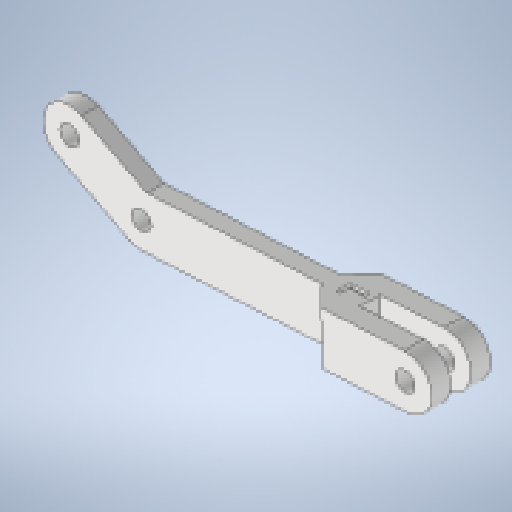
# Autodesk Inventor part: GripperShaftLeft
Saved by Autodesk Inventor 2025.1 (Build 291241000, 241)
## iProperties
Created: 2026-05-06
Part Number: GripperShaftLeft
Material: Generic
Document SubType Name: Modeling
Designer: User
Density: 1 g/cm^3
Appearance: Default
Author: User
## iProperties of the stored document GripperShaftLeft_3DPrint.ipt
Created: 2026-05-06
Part Number: GripperShaftLeft_3DPrint
Material: Generic
Document SubType Name: Modeling
Designer: User
Density: 1 g/cm^3
Appearance: Default
Author: User
Autodesk Inventor part; units mm, degrees
ref_plane "YZ Plane" through (0, 0, 0) normal (1, 0, 0) x (0, 1, 0)
ref_plane "XZ Plane" through (0, 0, 0) normal (0, 1, 0) x (-1, 0, 0)
sketch "Sketch1" plane through (0, 0, 0) normal (0, 0, 1) x (1, 0, 0)
  line L0 (-26.293304, 15.205533) -> (-26.696935, 23.195344)
  line L1 (-26.696935, 23.195344) -> (-13.921595, 23.840732)
  arc A0 (-13.517964, 15.85092) -> (-13.921595, 23.840732) centre (-13.719779, 19.845826) ccw
  line L2 (-13.517964, 15.85092) -> (-26.293304, 15.205533)
  circle A1 centre (-13.719779, 19.845826) radius 1.5
  point P0 (0, 0)
sketch "Sketch1 outline for Extrusion1" plane through (0, 0, 0) normal (0, 0, 1) x (1, 0, 0)
  arc A0 (-13.517964, 15.85092) -> (-13.921595, 23.840732) centre (-13.719779, 19.845826) ccw
  line L0 (-26.293304, 15.205533) -> (-13.517964, 15.85092)
  line L1 (-13.921595, 23.840732) -> (-26.696935, 23.195344)
  line L2 (-26.696935, 23.195344) -> (-26.293304, 15.205533)
  circle A1 centre (-13.719779, 19.845826) radius 1.5
extrude "Extrusion1" add sketch "Sketch1 outline for Extrusion1" along normal blind 3
sketch "Sketch2" plane through (0, 0, 0) normal (0, 0, -1) x (-1, 0, 0)
  line L0 (23.700756, 23.346705) -> (23.297124, 15.356894)
  line L1 (26.696935, 23.195344) -> (26.293304, 15.205533)
  line L2 (13.921595, 23.840732) -> (26.696935, 23.195344)
  arc A0 (13.921595, 23.840732) -> (13.517964, 15.85092) centre (13.719779, 19.845826) ccw
  line L3 (26.293304, 15.205533) -> (13.517964, 15.85092)
  line L4 (26.696935, 23.195344) -> (26.293304, 15.205533)
  circle A1 centre (13.719779, 19.845826) radius 1.5
  point P0 (0, 0)
sketch "Sketch2 outline for Extrusion2" plane through (0, 0, 0) normal (0, 0, -1) x (-1, 0, 0)
  line L0 (23.297124, 15.356894) -> (26.293304, 15.205533)
  line L1 (23.700756, 23.346705) -> (23.297124, 15.356894)
  line L2 (26.696935, 23.195344) -> (23.700756, 23.346705)
  line L3 (26.293304, 15.205533) -> (26.696935, 23.195344)
extrude "Extrusion2" add sketch "Sketch2 outline for Extrusion2" along normal blind 3.1
sketch "Sketch3" plane through (0, 0, -3.1) normal (0, 0, -1) x (-1, 0, 0)
  line L0 (13.921595, 23.840732) -> (26.696935, 23.195344)
  line L1 (26.696935, 23.195344) -> (26.293304, 15.205533)
  line L2 (26.293304, 15.205533) -> (13.517964, 15.85092)
  arc A0 (13.921595, 23.840732) -> (13.517964, 15.85092) centre (13.719779, 19.845826) ccw
  circle A1 centre (13.719779, 19.845826) radius 1.5
  point P0 (0, 0)
sketch "Sketch3 outline for Extrusion3" plane through (0, 0, -3.1) normal (0, 0, -1) x (-1, 0, 0)
  arc A0 (13.921595, 23.840732) -> (13.517964, 15.85092) centre (13.719779, 19.845826) ccw
  line L0 (26.696935, 23.195344) -> (13.921595, 23.840732)
  line L1 (13.517964, 15.85092) -> (26.293304, 15.205533)
  line L2 (26.293304, 15.205533) -> (26.696935, 23.195344)
  circle A1 centre (13.719779, 19.845826) radius 1.5
extrude "Extrusion3" add sketch "Sketch3 outline for Extrusion3" along normal blind 3
sketch "Sketch4" plane through (0, 0, 0) normal (0, 0, -1) x (-1, 0, 0)
  arc A0 (57.453567, 13.631371) -> (57.857198, 21.621182) centre (57.655383, 17.626276) ccw
  line L0 (57.453567, 13.631371) -> (29.389355, 15.049125)
  line L1 (29.792987, 23.038937) -> (29.389355, 15.049125)
  line L2 (29.792987, 23.038937) -> (57.857198, 21.621182)
  circle A1 centre (57.655383, 17.626276) radius 1.5
  line L3 (29.389355, 15.049125) -> (26.293304, 15.205533)
  line L4 (26.696935, 23.195344) -> (26.293304, 15.205533)
  line L5 (26.696935, 23.195344) -> (29.792987, 23.038937)
  line L6 (29.792987, 23.038937) -> (29.389355, 15.049125)
  circle A2 centre (68.688702, 23.388615) radius 1.5
  arc A3 (70.540437, 19.843043) -> (66.836967, 26.934186) centre (68.688702, 23.388615) ccw
  line L7 (59.507118, 14.080705) -> (70.540437, 19.843043)
  arc A4 (57.453567, 13.631371) -> (57.857198, 21.621182) centre (57.655383, 17.626276) ccw
  line L8 (56.769238, 21.676144) -> (66.836967, 26.934186)
  point P0 (0, 0)
  dimension "d18" = 8
  constraints: 6 end point, 5 point on circle, 4 tangent, 2 centre point, 2 coincident, 1 concentric, 1 point on line
  measures "d18" diameter of A3
sketch "Sketch4 outline for Extrusion4" plane through (0, 0, 0) normal (0, 0, -1) x (-1, 0, 0)
  line L0 (26.696935, 23.195344) -> (26.293304, 15.205533)
  line L1 (26.293304, 15.205533) -> (57.453567, 13.631371)
  arc A0 (57.453567, 13.631371) -> (59.507118, 14.080705) centre (57.655383, 17.626276) ccw
  line L2 (59.507118, 14.080705) -> (70.540437, 19.843043)
  arc A1 (70.540437, 19.843043) -> (66.836967, 26.934186) centre (68.688702, 23.388615) ccw
  line L3 (66.836967, 26.934186) -> (56.769238, 21.676144)
  line L4 (56.769238, 21.676144) -> (26.696935, 23.195344)
  circle A2 centre (57.655383, 17.626276) radius 1.5
  circle A3 centre (68.688702, 23.388615) radius 1.5
extrude "Extrusion4" add sketch "Sketch4 outline for Extrusion4" along normal blind 3
chamfer "Chamfer1" distance 3 angle 45 1 edges at (-26.4951, 19.2004, 0)
chamfer "Chamfer2" distance 3.1 angle 45 1 edges at (-26.4951, 19.2004, -3)
ref_plane "Work Plane1" through (-62.942605, 1.312432, -0.38873) normal (0, 0, -1) x (-0.0504539, 0.9987264, 0)
sketch "Sketch6" plane through (0, 0, 0) normal (0, 0, 1) x (1, 0, 0)
  line L0 (-57.453567, 13.631371) -> (-48.265284, 14.095547)
  arc A0 (-57.857198, 21.621182) -> (-57.453567, 13.631371) centre (-57.655383, 17.626276) ccw
  line L1 (-29.693114, 23.043982) -> (-57.857198, 21.621182)
  line L2 (-29.693114, 23.043982) -> (-48.265284, 14.095547)
  circle A1 centre (-57.655383, 17.626276) radius 1.5
  point P0 (0, 0)
sketch "Sketch6 outline for Extrusion5" plane through (0, 0, 0) normal (0, 0, 1) x (1, 0, 0)
  line L0 (-29.693114, 23.043982) -> (-57.857198, 21.621182)
  line L1 (-48.265284, 14.095547) -> (-29.693114, 23.043982)
  arc A0 (-57.857198, 21.621182) -> (-57.453567, 13.631371) centre (-57.655383, 17.626276) ccw
  line L2 (-57.453567, 13.631371) -> (-48.265284, 14.095547)
  circle A1 centre (-57.655383, 17.626276) radius 1.5
extrude "Extrusion5" cut sketch "Sketch6 outline for Extrusion5" against normal up to surface (0.38873 mm away)
sketch "Sketch7" plane through (-13.921595, 23.840732, 3) normal (-0.0504539, 0.9987264, 0) x (0.9987264, 0.0504539, 0)
  line L0 (-10.748057, 5.806776) -> (-10.748057, 3.406816) construction
  line L1 (-10.748057, 3.406816) -> (-13.798057, 3.406816) construction
  line L2 (-13.798057, 3.406816) -> (-13.798057, 5.806776) construction
  line L3 (-13.798057, 5.806776) -> (-10.748057, 5.806776) construction
  line L4 (-13.798057, 3.456249) -> (-13.798057, 5.490406)
  line L5 (-13.798057, 5.490406) -> (-10.748057, 5.490406)
  line L6 (-10.748057, 5.490406) -> (-10.748057, 4.724199)
  line L7 (-10.748057, 4.724199) -> (-13.217222, 4.724199)
  line L8 (-13.217222, 4.724199) -> (-13.217222, 3.456249)
  line L9 (-13.217222, 3.456249) -> (-13.798057, 3.456249)
  point P0 (12.701006, 3)
  constraints: 2 other
sketch "Sketch7 outline for Emboss1" plane through (-13.921595, 23.840732, 3) normal (-0.0504539, 0.9987264, 0) x (0.9987264, 0.0504539, 0)
  line L0 (-13.798057, 3.456249) -> (-13.798057, 5.490406)
  line L1 (-13.798057, 5.490406) -> (-10.748057, 5.490406)
  line L2 (-10.748057, 5.490406) -> (-10.748057, 4.724199)
  line L3 (-10.748057, 4.724199) -> (-13.217222, 4.724199)
  line L4 (-13.217222, 4.724199) -> (-13.217222, 3.456249)
  line L5 (-13.217222, 3.456249) -> (-13.798057, 3.456249)
emboss "Emboss1" sketch "Sketch7 outline for Emboss1" operation cut depth 0.5 direction (0.0504539, -0.9987264, 0)
sketch "Sketch8" plane through (0, 0, 0) normal (0, 0, 1) x (1, 0, 0)
  line L0 (-57.857198, 21.621182) -> (-56.769238, 21.676144)
  line L1 (-66.836967, 26.934186) -> (-56.769238, 21.676144)
  arc A0 (-66.836967, 26.934186) -> (-70.540437, 19.843043) centre (-68.688702, 23.388615) ccw
  line L2 (-59.507118, 14.080705) -> (-70.540437, 19.843043)
  arc A1 (-57.857198, 21.621182) -> (-59.507118, 14.080705) centre (-57.655383, 17.626276) ccw
  circle A2 centre (-68.688702, 23.388615) radius 1.5
  point P0 (0, 0)
sketch "Sketch8 outline for Extrusion6" plane through (0, 0, 0) normal (0, 0, 1) x (1, 0, 0)
  arc A0 (-59.507118, 14.080705) -> (-57.857198, 21.621182) centre (-57.655383, 17.626276) cw
  line L0 (-70.540437, 19.843043) -> (-59.507118, 14.080705)
  line L1 (-57.857198, 21.621182) -> (-56.769238, 21.676144)
  arc A1 (-66.836967, 26.934186) -> (-70.540437, 19.843043) centre (-68.688702, 23.388615) ccw
  line L2 (-56.769238, 21.676144) -> (-66.836967, 26.934186)
  circle A2 centre (-68.688702, 23.388615) radius 1.5
extrude "Extrusion6" cut sketch "Sketch8 outline for Extrusion6" against normal up to surface (0.38873 mm away)
sketch "Sketch9" plane through (0, 0, 0) normal (0, 0, 1) x (1, 0, 0)
  line L0 (-29.693114, 23.043982) -> (-48.265284, 14.095547)
  line L1 (-29.289483, 15.054171) -> (-48.265284, 14.095547)
  line L2 (-29.693114, 23.043982) -> (-29.289483, 15.054171)
  point P0 (0, 0)
sketch "Sketch9 outline for Extrusion7" plane through (0, 0, 0) normal (0, 0, 1) x (1, 0, 0)
  line L0 (-29.289483, 15.054171) -> (-29.693114, 23.043982)
  line L1 (-48.265284, 14.095547) -> (-29.289483, 15.054171)
  line L2 (-29.693114, 23.043982) -> (-48.265284, 14.095547)
extrude "Extrusion7" cut sketch "Sketch9 outline for Extrusion7" against normal up to surface (0.38873 mm away)
body "Solid1"
